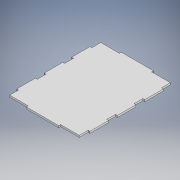
# Autodesk Inventor part: Placa de abajo
Saved by Autodesk Inventor 2020 (Build 240168000, 168)
## iProperties
Created: 2020-03-11
Part Number: Placa de abajo
Material: Generic
Document SubType Name: Modeling
Designer: José Javier Estrada
Density: 1 g/cm^3
Appearance: Default
Author: José Javier Estrada
Autodesk Inventor part; units mm, degrees
ref_plane "YZ Plane" through (0, 0, 0) normal (1, 0, 0) x (0, 1, 0)
ref_plane "XZ Plane" through (0, 0, 0) normal (0, 1, 0) x (-1, 0, 0)
ref_plane "XY Plane" through (0, 0, 0) normal (0, 0, 1) x (1, 0, 0)
sketch "Sketch1" plane through (0, 0, 0) normal (0, 1, 0) x (-1, 0, 0)
  line L0 (0, 0) -> (187, 0)
  line L1 (187, 0) -> (187, -245)
  line L2 (187, -245) -> (0, -245)
  line L3 (0, -245) -> (0, 0)
  dimension "d0" = 245
  dimension "d1" = 187
  constraints: 8 end point, 2 parallel, 1 horizontal, 1 perpendicular
  measures "d0" distance of L0.end L1.end
  measures "d1" distance of L1.end L2.end
extrude "Extrusion1" add sketch "Sketch1" along normal blind 5
sketch "Sketch2" plane through (0, 5, 0) normal (0, 1, 0) x (1, 0, 0)
  line L0 (-187, 0) -> (0, 0) projected
  line L1 (0, 0) -> (0, 245) projected
  line L2 (0, 245) -> (-187, 245) projected
  line L3 (-187, 245) -> (-187, 0) projected
  line L4 (-187, 221.25) -> (-192, 221.25)
  line L5 (-192, 221.25) -> (-192, 171.25)
  line L6 (-192, 171.25) -> (-187, 171.25)
  line L7 (-187, 171.25) -> (-187, 221.25)
  line L8 (-192, 147.5) -> (-187, 147.5)
  line L9 (-187, 147.5) -> (-187, 97.5)
  line L10 (-187, 97.5) -> (-192, 97.5)
  line L11 (-192, 97.5) -> (-192, 147.5)
  line L12 (-192, 73.75) -> (-187, 73.75)
  line L13 (-187, 73.75) -> (-187, 23.75)
  line L14 (-187, 23.75) -> (-192, 23.75)
  line L15 (-192, 23.75) -> (-192, 73.75)
  line L16 (5, 221.25) -> (0, 221.25)
  line L17 (0, 221.25) -> (0, 171.25)
  line L18 (0, 171.25) -> (5, 171.25)
  line L19 (5, 171.25) -> (5, 221.25)
  line L20 (0, 147.5) -> (5, 147.5)
  line L21 (5, 147.5) -> (5, 97.5)
  line L22 (5, 97.5) -> (0, 97.5)
  line L23 (0, 97.5) -> (0, 147.5)
  line L24 (0, 73.75) -> (5, 73.75)
  line L25 (5, 73.75) -> (5, 23.75)
  line L26 (5, 23.75) -> (0, 23.75)
  line L27 (0, 23.75) -> (0, 73.75)
  line L28 (-137, 250) -> (-50, 250)
  line L29 (-50, 250) -> (-50, 245)
  line L30 (-50, 245) -> (-137, 245)
  line L31 (-137, 245) -> (-137, 250)
  line L32 (-137, 0) -> (-50, 0)
  line L33 (-50, 0) -> (-50, -5)
  line L34 (-50, -5) -> (-137, -5)
  line L35 (-137, -5) -> (-137, 0)
  point P0 (-50, 0)
  dimension "d4" = 5
  dimension "d5" = 50
  dimension "d6" = 50
  dimension "d7" = 50
  dimension "d8" = 5
  dimension "d9" = 5
  dimension "d10" = 23.75
  dimension "d11" = 23.75
  dimension "d12" = 23.75
  dimension "d13" = 5
  dimension "d14" = 50
  dimension "d15" = 50
  dimension "d16" = 50
  dimension "d17" = 5
  dimension "d18" = 5
  dimension "d19" = 23.75
  dimension "d20" = 23.75
  dimension "d21" = 23.75
  dimension "d22" = 5
  dimension "d23" = 50
  dimension "d24" = 50
  dimension "d25" = 5
  dimension "d26" = 50
  dimension "d27" = 50
  constraints: 64 end point, 16 parallel, 8 horizontal, 8 perpendicular, 7 collinear, 1 point on line
  measures "d4" distance of L4.start L4.end
  measures "d5" distance of L4.end L5.end
  measures "d6" distance of L14.end L12.start
  measures "d7" distance of L10.end L8.start
  measures "d8" distance of L8.start L8.end
  measures "d9" distance of L12.start L12.end
  measures "d10" distance between parallel lines of L2 L4
  measures "d11" distance between parallel lines of L6 L8
  measures "d12" distance between parallel lines of L10 L12
  measures "d13" distance of L19.end L17.start
  measures "d14" distance of L17.start L18.start
  measures "d15" distance of L27.start L24.start
  measures "d16" distance of L23.start L23.end
  measures "d17" distance of L23.end L21.start
  measures "d18" distance of L24.start L24.end
  measures "d19" distance between parallel lines of L18 L20
  measures "d20" distance between parallel lines of L22 L24
  measures "d21" distance between parallel lines of L2 L16
  measures "d22" distance of L28.end L29.end
  measures "d23" distance between parallel lines of L1 L29
  measures "d24" distance between parallel lines of L3 L31
  measures "d25" distance of L32.end L34.start
  measures "d26" distance between parallel lines of L3 L35
  measures "d27" distance between parallel lines of L1 L33
extrude "Extrusion2" add sketch "Sketch2" against normal blind 5 contours L0 L33 L34 L35 | L14 L15 L12 L3 | L10 L11 L8 L3 | L1 L24 L25 L26 | L6 L5 L4 L3 | L1 L20 L21 L22 | L1 L16 L19 L18 | L31 L28 L29 L2
body "Solid1"
